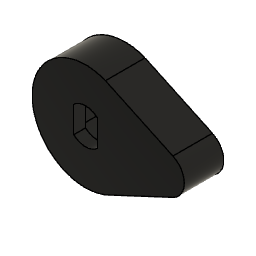
1-90_Cam (Autodesk Fusion 360 design; units mm, degrees)
Autodesk Fusion 360 part; units mm, degrees
sketch "Sketch1" plane through (0, 0, 0) normal (0, 1, 0) x (1, 0, 0)
  arc A0 (-2, -13.1375) -> (2, -13.1375) centre (0, -11.25) ccw
  line L0 (-2, -13.1375) -> (-2, -9.3625)
  arc A1 (2, -9.3625) -> (-2, -9.3625) centre (0, -11.25) ccw
  line L1 (2, -9.3625) -> (2, -13.1375)
  line L2 (-2.5, -13.3267) -> (-2.5, -9.1733)
  arc A2 (2.5, -9.1733) -> (-2.5, -9.1733) centre (0, -11.25) ccw
  line L3 (2.5, -9.1733) -> (2.5, -13.3267)
  arc A3 (-2.5, -13.3267) -> (2.5, -13.3267) centre (0, -11.25) ccw
  arc A4 (-6, -14.3423) -> (6, -14.3423) centre (0, -11.25) ccw
  line L4 (6, -8.1577) -> (6, -14.3423)
  arc A5 (6, -8.1577) -> (-6, -8.1577) centre (0, -11.25) ccw
  line L5 (-6, -14.3423) -> (-6, -8.1577)
  circle A6 centre (10, -11.25) radius 2.5
  line L6 (2.5219, -17.5112) -> (11.06, -13.5142)
  line L7 (3.1933, -5.3031) -> (11.06, -8.9858)
  line L8 (1.5, -9.5729) -> (1.5, -12.9271)
  arc A7 (-1.5, -12.9271) -> (1.5, -12.9271) centre (0, -11.25) ccw
  line L9 (-1.5, -12.9271) -> (-1.5, -9.5729)
  arc A8 (1.5, -9.5729) -> (-1.5, -9.5729) centre (0, -11.25) ccw
  circle A9 centre (0, -11.25) radius 6.75
  dimension "d1" = 0.5
  dimension "d2" = -4
  dimension "d3" = 5
  dimension "d4" = 10
  dimension "d7" = 0.5
  dimension "d10" = 13.5
  constraint coincident A4 L6.start
  constraint coincident A6 L6.end
  constraint tangent A6 L6
  constraint coincident A5 L7.start
  constraint coincident A6 L7.end
  constraint tangent A6 L7
  constraint concentric A1 A9
  measures "d3" diameter of A6
  measures "d4" distance of A0.centre A6.centre
  measures "d10" diameter of A9
extrude "Extrude1" add sketch "Sketch1" along normal blind 5 contours A4 L4 A5 L5 L6 A9 | L5 A9 | A4 A5 A6 L6 L7 A9 | L4 A9 | A6
extrude "Extrude2" add sketch "Sketch1" along normal blind 1.5 contours A0 L0 A1 L1 | L2 A2 L3 A3
